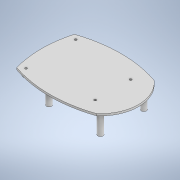
# Autodesk Inventor part: 06_RPLidar_Raspi_Adabter
Saved by Autodesk Inventor 2021 (Build 250183000, 183)
## iProperties
Created: 2021-06-05
Part Number: 06_RPLidar_Raspi_Adabter
Material: Generisch
Document SubType Name: Modeling
Designer: User
Density: 1 g/cm^3
Appearance: Vorgabe
Author: User
## iProperties of the stored document _3D-Druck.ipt
Created: 2021-06-06
Part Number: _3D-Druck
Material: Generisch
Document SubType Name: Modeling
Designer: User
Density: 1 g/cm^3
Appearance: Vorgabe
Author: User
Autodesk Inventor part; units mm, degrees
ref_plane "YZ Plane" through (0, 0, 0) normal (1, 0, 0) x (0, 1, 0)
ref_plane "XZ Plane" through (0, 0, 0) normal (0, 1, 0) x (-1, 0, 0)
sketch "Skizze4" plane through (0, 0, 0) normal (0, 1, 0) x (-1, 0, 0)
  arc A0 (45, -32.5) -> (45, 32.5) centre (-70.5152, 0) ccw
  arc A1 (45, 32.5) -> (-45, 32.5) centre (0, -98.75) ccw
  arc A2 (-45, 32.5) -> (-45, -32.5) centre (-16.8442, 0) ccw
  line L0 (49.4848, 0) -> (-59.8442, 0) construction
  circle A3 centre (39, -28) radius 1.225
  circle A4 centre (39, 28) radius 1.225
  circle A5 centre (-31, 20) radius 1.225
  circle A6 centre (-31, -20) radius 1.225
  circle A7 centre (16.53, -24.5) radius 1.225
  circle A8 centre (16.53, 24.5) radius 1.225
  circle A9 centre (-41.47, 24.5) radius 1.225
  circle A10 centre (-41.47, -24.5) radius 1.225
  line L1 (39, 28) -> (39, -28) construction
  line L2 (39, -28) -> (-31, -20) construction
  line L3 (-31, -20) -> (-31, 20) construction
  line L4 (-31, 20) -> (39, 28) construction
  line L5 (16.53, 24.5) -> (16.53, -24.5) construction
  line L6 (16.53, -24.5) -> (-41.47, -24.5) construction
  line L7 (-41.47, -24.5) -> (-41.47, 24.5) construction
  line L8 (-41.47, 24.5) -> (16.53, 24.5) construction
  line L9 (0, -40) -> (0, 40) construction
  circle A11 centre (16.53, -24.5) radius 2.9
  circle A12 centre (-41.47, -24.5) radius 2.9
  circle A13 centre (-41.47, 24.5) radius 2.9
  circle A14 centre (16.53, 24.5) radius 2.9
  line L10 (45, 32.5) -> (45, -32.5) construction
  line L11 (-45, 32.5) -> (-45, -32.5) construction
  arc A15 (-45, -32.5) -> (45, -32.5) centre (0, 98.75) ccw
  circle A16 centre (-31, -20) radius 3
  circle A17 centre (-31, 20) radius 3
  circle A18 centre (39, 28) radius 3
  circle A19 centre (39, -28) radius 3
  point P0 (0, 0)
  point P1 (0, 0)
  dimension "d19" = 2.45
  dimension "d20" = 5.8
  dimension "d28" = 80
  dimension "d30" = 90
  dimension "d31" = 58
  dimension "d32" = 49
  dimension "d33" = 56
  dimension "d34" = 40
  dimension "d35" = 70
  dimension "d36" = 65
  dimension "d37" = 65
  dimension "d38" = 22.47
  dimension "d39" = 120
  dimension "d40" = 6
  dimension "d41" = 2.45
  dimension "d42" = 43
  dimension "d58" = 6
  constraints: 24 end point, 20 centre point, 13 equal radius, 12 point on circle, 9 coincident, 7 perpendicular, 2 parallel, 1 midpoint, 1 point on line, 1 vertical, 2 other
  measures "d19" diameter of A7
  measures "d20" diameter of A11
  measures "d28" distance of L9.start L9.end
  measures "d30" distance between parallel lines of L10 L11
  measures "d31" distance between parallel lines of L5 L7
  measures "d32" distance of L6.end L7.end
  measures "d33" distance of L1.start L1.end
  measures "d34" distance of L2.end L3.end
  measures "d35" distance between parallel lines of L1 L3
  measures "d36" distance of L10.start L10.end
  measures "d37" distance of L11.start L11.end
  measures "d38" distance between parallel lines of L1 L5
  measures "d39" radius of A0
  measures "d40" distance from line of L1 L10.end
  measures "d41" diameter of A3
  measures "d42" radius of A2
  measures "d58" diameter of A19
sketch "Skizze3" plane through (0, 0, 0) normal (0, 1, 0) x (-1, 0, 0)
  line L0 (-220.6772, -144.4743) -> (-220.6772, -104.4743)
  line L1 (-220.6772, -104.4743) -> (-150.6772, -96.4743)
  line L2 (-150.6772, -96.4743) -> (-150.6772, -152.4743)
  line L3 (-150.6772, -152.4743) -> (-220.6772, -144.4743)
  line L4 (-173.154, -148.9743) -> (-231.154, -148.9743)
  line L5 (-231.154, -148.9743) -> (-231.154, -99.9743)
  line L6 (-231.154, -99.9743) -> (-173.154, -99.9743)
  line L7 (-173.154, -99.9743) -> (-173.154, -148.9743)
  circle A0 centre (-231.154, -99.9743) radius 1.35
  circle A1 centre (-231.154, -148.9743) radius 1.35
  circle A2 centre (-173.154, -148.9743) radius 1.35
  circle A3 centre (-173.154, -99.9743) radius 1.35
  arc A4 (-234.6505, -110.3469) -> (-234.6486, -138.3994) centre (-219.7787, -124.3722) ccw
  line L8 (-234.6505, -110.3469) -> (-234.6458, -99.4805)
  arc A5 (-231.5992, -96.4365) -> (-234.6458, -99.4805) centre (-231.6005, -99.4818) ccw
  line L9 (-231.5992, -96.4365) -> (-212.1876, -96.4449)
  arc A6 (-178.6836, -89.0505) -> (-212.1876, -96.4449) centre (-176.7514, -177.4047) ccw
  arc A7 (-149.827, -93.1805) -> (-178.6836, -89.0505) centre (-181.982, -214.9715) ccw
  arc A8 (-147.411, -95.6063) -> (-149.827, -93.1805) centre (-150.6924, -96.4584) ccw
  arc A9 (-143.2995, -124.3735) -> (-147.411, -95.6063) centre (-273.1451, -128.2544) ccw
  arc A10 (-147.4215, -153.3903) -> (-143.2995, -124.3735) centre (-273.1519, -120.7284) ccw
  arc A11 (-149.7866, -155.739) -> (-147.4215, -153.3903) centre (-150.6843, -152.4698) ccw
  arc A12 (-178.6402, -159.8288) -> (-149.7866, -155.739) centre (-181.7729, -33.9036) ccw
  arc A13 (-212.2336, -152.5079) -> (-178.6402, -159.8288) centre (-176.9785, -71.4691) ccw
  line L10 (-231.6452, -152.4995) -> (-212.2336, -152.5079)
  arc A14 (-234.6534, -149.2659) -> (-231.6452, -152.4995) centre (-231.6139, -149.4543) ccw
  line L11 (-234.6534, -149.2659) -> (-234.6486, -138.3994)
  line L12 (-240.2208, -124.3735) -> (-143.2995, -124.3735) construction
  line L13 (-177.3977, -89.0907) -> (-177.3977, -159.7918) construction
  point P0 (-177.3977, -124.4413)
  constraints: 28 end point, 25 point on circle, 15 centre point, 6 perpendicular, 5 equal radius, 4 parallel, 4 tangent, 1 horizontal, 1 midpoint, 1 vertical
extrude "Extrusion1" add sketch "Skizze4" along normal blind 2.2 contours A15 A2 A1 A0 | A7 | A8 | A9 | A10 | A11 | A12 | A13 | A14 | A16 | A17 | A18 | A19
extrude "Extrusion2" add sketch "Skizze4" against normal blind 24 contours A11 | A12 | A13 | A14
extrude "Extrusion3" add sketch "Skizze4" against normal blind 5 contours A16 | A17 | A18 | A19
ref_plane "Arbeitsebene1" through (41.47, 0, -24.5) normal (-0.3949, 0, -0.9187) x (0, -1, 0)
sketch "Skizze6" plane through (41.47, 0, -24.5) normal (-0.3949, 0, -0.9187) x (0, -1, 0)
  line L0 (24, 1.2564) -> (24.1406, 1.5)
  line L1 (24.1406, 1.5) -> (24.1969, 1.5)
  line L2 (24.1969, 1.5) -> (24.3375, 1.2564)
  line L3 (24.3375, 1.2564) -> (24.3937, 1.2564)
  line L4 (24.45, 1.2564) -> (24.45, 1.5487) construction
  line L5 (24.45, 1.5487) -> (23.8875, 1.5487) construction
  line L6 (23.8875, 1.5487) -> (23.8875, 1.2564) construction
  line L7 (23.8875, 1.2564) -> (23.9437, 1.2564) construction
  line L8 (23.9437, 1.2564) -> (24, 1.2564)
  line L9 (24.3937, 1.2564) -> (24.45, 1.2564) construction
  line L10 (24, 1.2564) -> (24.3375, 1.2564) construction
  line L11 (24.1406, 1.5) -> (24.1687, 1.5487) construction
  line L12 (24.1969, 1.5) -> (24.1687, 1.5487) construction
  line L13 (23.8875, 0) -> (24.45, 0) construction
  line L14 (23.8875, 1.2564) -> (23.9437, 1.159) construction
  line L15 (23.9437, 1.159) -> (24, 1.2564) construction
  line L16 (24.3375, 1.2564) -> (24.3937, 1.159) construction
  line L17 (24.3937, 1.159) -> (24.45, 1.2564) construction
  line L18 (24.1687, 1.2564) -> (24.1687, 1.5487) construction
  line L19 (23.9437, 1.159) -> (24.3937, 1.159) construction
  line L20 (23.8875, 0) -> (23.8875, 1.2564) construction
  line L21 (24.45, 0) -> (24.45, 1.2564) construction
  line L22 (-7.98, 0) -> (29.33, 0) projected
  line L23 (24, 1.225) -> (24, -1.225) projected
  line L24 (24, 1.2564) -> (24.3375, 1.2564)
  line L25 (-2.5375, 12.6525) -> (-2.3969, 12.8961)
  line L26 (-2.3969, 12.8961) -> (-2.3406, 12.8961)
  line L27 (-2.3406, 12.8961) -> (-2.2, 12.6525)
  line L28 (-2.2, 12.6525) -> (-2.1437, 12.6525)
  line L29 (-2.0875, 12.6525) -> (-2.0875, 12.9448) construction
  line L30 (-2.0875, 12.9448) -> (-2.65, 12.9448) construction
  line L31 (-2.65, 12.9448) -> (-2.65, 12.6525) construction
  line L32 (-2.65, 12.6525) -> (-2.5937, 12.6525) construction
  line L33 (-2.5937, 12.6525) -> (-2.5375, 12.6525)
  line L34 (-2.1437, 12.6525) -> (-2.0875, 12.6525) construction
  line L35 (-2.5375, 12.6525) -> (-2.2, 12.6525) construction
  line L36 (-2.3969, 12.8961) -> (-2.3687, 12.9448) construction
  line L37 (-2.3406, 12.8961) -> (-2.3687, 12.9448) construction
  line L38 (-2.65, 11.3961) -> (-2.0875, 11.3961) construction
  line L39 (-2.65, 12.6525) -> (-2.5937, 12.5551) construction
  line L40 (-2.5937, 12.5551) -> (-2.5375, 12.6525) construction
  line L41 (-2.2, 12.6525) -> (-2.1437, 12.5551) construction
  line L42 (-2.1437, 12.5551) -> (-2.0875, 12.6525) construction
  line L43 (-2.3687, 12.6525) -> (-2.3687, 12.9448) construction
  line L44 (-2.5937, 12.5551) -> (-2.1437, 12.5551) construction
  line L45 (-2.65, 11.3961) -> (-2.65, 12.6525) construction
  line L46 (-2.0875, 11.3961) -> (-2.0875, 12.6525) construction
  line L47 (29.33, 11.3961) -> (-7.98, 11.3961) projected
  line L48 (-2.5375, 12.6525) -> (-2.2, 12.6525)
  line L49 (-2.2, 10.1711) -> (-2.2, 12.6211) projected
  dimension "d47" = 60
  dimension "d48" = 3
  dimension "d49" = 0.45
  dimension "d50" = 2.5129
  dimension "d51" = 0.2436
  dimension "d52" = 0.0487
  dimension "d62" = 0
  dimension "d71" = 60
  dimension "d72" = 3
  dimension "d73" = 0.45
  dimension "d74" = 2.5129
  dimension "d75" = 0.2436
  dimension "d76" = 0.0487
  dimension "d82" = 0
  constraints: 92 end point, 22 collinear, 10 parallel, 6 midpoint, 6 perpendicular, 4 coincident, 4 point on line, 18 other
  measures "d47" angle of L0 L2
  measures "d48" diameter of L0.end L13
  measures "d49" distance of L7.end L3.end
  measures "d50" diameter of L7.end L13
  measures "d51" distance between parallel lines of L1 L10
  measures "d52" distance from line of L18.end L1
  measures "d62" distance from line of L23 L0.start
  measures "d71" angle of L25 L27
  measures "d72" diameter of L25.end L38
  measures "d73" distance of L32.end L28.end
  measures "d74" diameter of L32.end L38
  measures "d75" distance between parallel lines of L26 L35
  measures "d76" distance from line of L43.end L26
  measures "d82" distance from line of L28.start L49
equation "\"d53\" = 60deg"
equation "\"d54\" = 3"
equation "\"d55\" = 0.45"
equation "\"d56\" = 2.51288"
equation "\"d57\" = 0.3897"
equation "\"d77\" = 60deg"
equation "\"d78\" = 3"
equation "\"d79\" = 0.45"
equation "\"d80\" = 2.51288"
equation "\"d81\" = 0.3897"
